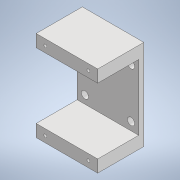
# Autodesk Inventor part: bearingV2
Saved by Autodesk Inventor 2022 (Build 260153000, 153)
## iProperties
Created: 2022-05-04
Part Number: bearingV2
Material: Generic
Document SubType Name: Modeling
Designer: erasm
Density: 1 g/cm^3
Appearance: Default
Author: erasm
Autodesk Inventor part; units mm, degrees
ref_plane "YZ Plane" through (0, 0, 0) normal (1, 0, 0) x (0, 1, 0)
ref_plane "XZ Plane" through (0, 0, 0) normal (0, 1, 0) x (-1, 0, 0)
ref_plane "XY Plane" through (0, 0, 0) normal (0, 0, 1) x (1, 0, 0)
sketch "Sketch1" plane through (0, 0, 0) normal (0, 0, 1) x (1, 0, 0)
  line L0 (-30, 44) -> (-30, -44) projected
  line L1 (-30, -44) -> (30, -44) projected
  line L2 (30, -44) -> (30, 44) projected
  line L3 (30, 44) -> (-30, 44) projected
  circle A0 centre (22.5, -24) radius 3 projected
  circle A1 centre (-22.5, -24) radius 3 projected
  line L4 (-15, -4) -> (-30, -4) projected
  line L5 (-30, -4) -> (-30, -44) projected
  line L6 (-15, -44) -> (-30, -44) projected
  line L7 (-15, -4) -> (-15, -44) projected
  circle A2 centre (-22.5, 24) radius 3 projected
  line L8 (-15, 44) -> (-30, 44) projected
  line L9 (-30, 44) -> (-30, 4) projected
  line L10 (-15, 4) -> (-30, 4) projected
  line L11 (-15, 44) -> (-15, 4) projected
  circle A3 centre (-22.5, 24) radius 3 projected
  line L12 (-15, 4) -> (-30, 4) projected
  line L13 (-30, 4) -> (-30, 44) projected
  line L14 (-15, 44) -> (-30, 44) projected
  line L15 (-15, 4) -> (-15, 44) projected
  circle A4 centre (-22.5, 24) radius 3 projected
  line L16 (-15, 4) -> (-30, 4) projected
  line L17 (-30, 4) -> (-30, 44) projected
  line L18 (-15, 44) -> (-30, 44) projected
  line L19 (-15, 4) -> (-15, 44) projected
  circle A5 centre (-22.5, 24) radius 3 projected
  line L20 (-15, 4) -> (-30, 4) projected
  line L21 (-30, 4) -> (-30, 44) projected
  line L22 (-15, 44) -> (-30, 44) projected
  line L23 (-15, 4) -> (-15, 44) projected
  circle A6 centre (-22.5, 24) radius 3 projected
  line L24 (-15, 4) -> (-30, 4) projected
  line L25 (-30, 4) -> (-30, 44) projected
  line L26 (-15, 44) -> (-30, 44) projected
  line L27 (-15, 4) -> (-15, 44) projected
  circle A7 centre (-22.5, 24) radius 3 projected
  line L28 (-15, 4) -> (-30, 4) projected
  line L29 (-30, 4) -> (-30, 44) projected
  line L30 (-15, 44) -> (-30, 44) projected
  line L31 (-15, 4) -> (-15, 44) projected
  circle A8 centre (22.5, 24) radius 3 projected
  line L32 (30, 4) -> (15, 4) projected
  line L33 (15, 4) -> (15, 44) projected
  line L34 (30, 44) -> (15, 44) projected
  line L35 (30, 4) -> (30, 44) projected
  point P0 (0, 0)
extrude "Extrusion1" add sketch "Sketch1" along normal blind 5
sketch "Sketch2" plane through (0, 0, 5) normal (0, 0, 1) x (1, 0, 0)
  line L0 (30, 44) -> (-30, 44) projected
  line L1 (-30, 44) -> (-30, -44) projected
  line L2 (30, 44) -> (-30, 44)
  line L3 (-30, 44) -> (-30, 32)
  line L4 (-30, 32) -> (30, 32)
  line L5 (30, 32) -> (30, 44)
  line L6 (30, -44) -> (-30, -44)
  line L7 (-30, -44) -> (-30, -32)
  line L8 (-30, -32) -> (30, -32)
  line L9 (30, -32) -> (30, -44)
  point P0 (0, 0)
  dimension "d2" = 12
  dimension "d3" = 12
  constraints: 16 end point, 4 parallel, 2 horizontal, 2 perpendicular, 2 point on line
  measures "d2" distance between parallel lines of L0 L4
  measures "d3" distance of L6.end L7.end
extrude "Extrusion2" add sketch "Sketch2" along normal blind 40
sketch "Sketch3" plane through (0, 0, 45) normal (0, 0, 1) x (1, 0, 0)
  circle A0 centre (21, 38) radius 1.5
  circle A1 centre (-21, 38) radius 1.5
  circle A2 centre (21, -38) radius 1.5
  circle A3 centre (-21, -38) radius 1.5
  line L0 (-30, 32) -> (30, 32) projected
  line L1 (-30, -44) -> (30, -44) projected
  line L2 (30, 32) -> (30, 44) projected
  line L3 (30, -44) -> (30, -32) projected
  point P0 (0, 0)
  dimension "d6" = 3
  dimension "d7" = 3
  dimension "d8" = 3
  dimension "d9" = 3
  dimension "d10" = 6
  dimension "d11" = 6
  dimension "d12" = 42
  dimension "d13" = 42
  dimension "d14" = 9
  dimension "d15" = 9
  constraints: 4 centre point, 2 horizontal alignment
  measures "d6" diameter of A0
  measures "d7" diameter of A1
  measures "d8" diameter of A2
  measures "d9" diameter of A3
  measures "d10" distance from line of L0 A0.centre
  measures "d11" distance from line of L1 A2.centre
  measures "d12" distance of A1.centre A0.centre
  measures "d13" distance of A3.centre A2.centre
  measures "d14" distance from line of L2 A0.centre
  measures "d15" distance from line of L3 A2.centre
extrude "Extrusion3" cut sketch "Sketch3" against normal blind 5
sketch "Sketch4" plane through (0, 0, 5) normal (0, 0, 1) x (1, 0, 0)
  circle A0 centre (22.5, 24) radius 3 projected
  circle A1 centre (22.5, 24) radius 3.5
  circle A2 centre (22.5, -24) radius 3 projected
  circle A3 centre (22.5, -24) radius 3.5
  circle A4 centre (-22.5, 24) radius 3 projected
  circle A5 centre (-22.5, 24) radius 3.5
  circle A6 centre (-22.5, -24) radius 3 projected
  circle A7 centre (-22.5, -24) radius 3.5
  point P0 (0, 0)
  dimension "d18" = 7
  dimension "d19" = 7
  dimension "d20" = 7
  dimension "d21" = 7
  constraints: 4 centre point, 4 coincident
  measures "d18" diameter of A1
  measures "d19" diameter of A3
  measures "d20" diameter of A5
  measures "d21" diameter of A7
extrude "Extrusion4" cut sketch "Sketch4" against normal blind 5 contours A0 | A1 | A2 | A3 | A4 | A5 | A6 | A7
ref_plane "Work Plane1" through (0, -44, 0) normal (-1, 0, 0) x (0, 0, 1)
sketch "Sketch5" plane through (0, -44, 0) normal (-1, 0, 0) x (0, 0, 1)
  line L0 (5, 76) -> (5, 12) projected
  line L1 (5, 76) -> (5, 51)
  line L2 (45, 76) -> (45, 88) projected
  line L3 (5, 51) -> (45, 76)
  line L4 (5, 76) -> (45, 76) projected
  line L5 (45, 76) -> (5, 76)
  line L6 (5, 12) -> (45, 12) projected
  line L7 (5, 12) -> (5, 37)
  line L8 (45, 12) -> (45, 0) projected
  line L9 (5, 37) -> (45, 12)
  line L10 (45, 12) -> (5, 12)
  point P0 (0, 44)
  dimension "d24" = 25
  dimension "d25" = 25
  constraints: 12 end point, 2 point on line, 1 collinear, 1 perpendicular
  measures "d24" distance of L0.start L1.end
  measures "d25" distance of L0.end L7.end
extrude "Extrusion5" add sketch "Sketch5" along normal mid plane 12
body "Solid1"
